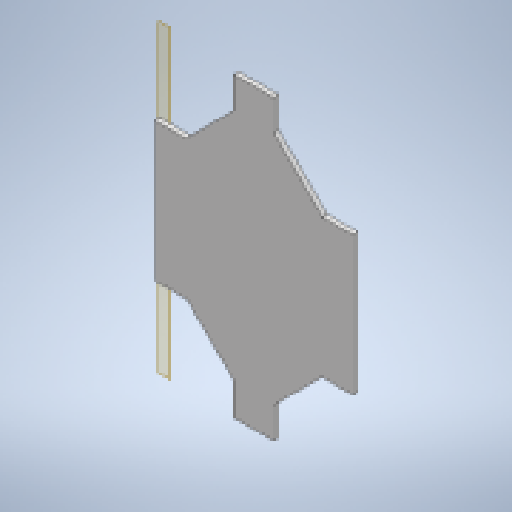
# Autodesk Inventor part: baseplate
Saved by Autodesk Inventor 2024 (Build 280153000, 153)
## iProperties
Created: 2024-01-06
Part Number: baseplate
Material: Generic
Document SubType Name: Modeling
Designer: student
Density: 1 g/cm^3
Appearance: Default
Author: student
Autodesk Inventor part; units mm, degrees
ref_plane "YZ Plane" through (0, 0, 0) normal (1, 0, 0) x (0, 1, 0)
ref_plane "XZ Plane" through (0, 0, 0) normal (0, 1, 0) x (-1, 0, 0)
ref_plane "XY Plane" through (0, 0, 0) normal (0, 0, 1) x (1, 0, 0)
ref_plane "Work Plane1" through (0, 0, 0) normal (0, 0, 1) x (1, 0, 0)
sketch "Sketch1" plane through (0, 0, 0) normal (0, 0, 1) x (1, 0, 0)
  circle A0 centre (495.3, 317.5) radius 1.5875
  circle A1 centre (495.3, 698.5) radius 1.5875
  circle A2 centre (495.3, 673.1) radius 1.5875
  circle A3 centre (495.3, 647.7) radius 1.5875
  circle A4 centre (495.3, 622.3) radius 1.5875
  circle A5 centre (495.3, 596.9) radius 1.5875
  circle A6 centre (495.3, 571.5) radius 1.5875
  circle A7 centre (495.3, 546.1) radius 1.5875
  circle A8 centre (495.3, 520.7) radius 1.5875
  circle A9 centre (495.3, 495.3) radius 1.5875
  circle A10 centre (495.3, 469.9) radius 1.5875
  circle A11 centre (495.3, 444.5) radius 1.5875
  circle A12 centre (495.3, 419.1) radius 1.5875
  circle A13 centre (495.3, 393.7) radius 1.5875
  circle A14 centre (495.3, 368.3) radius 1.5875
  circle A15 centre (495.3, 342.9) radius 1.5875
  circle A16 centre (495.3, 317.5) radius 1.5875
  circle A17 centre (495.3, 292.1) radius 1.5875
  circle A18 centre (495.3, 266.7) radius 1.5875
  circle A19 centre (495.3, 241.3) radius 1.5875
  circle A20 centre (495.3, 215.9) radius 1.5875
  circle A21 centre (495.3, 190.5) radius 1.5875
  circle A22 centre (495.3, 165.1) radius 1.5875
  circle A23 centre (495.3, 139.7) radius 1.5875
  circle A24 centre (495.3, 114.3) radius 1.5875
  circle A25 centre (495.3, 88.9) radius 1.5875
  circle A26 centre (495.3, 63.5) radius 1.5875
  circle A27 centre (495.3, 38.1) radius 1.5875
  circle A28 centre (495.3, 12.7) radius 1.5875
  line L0 (482.6, 0) -> (508, 0)
  line L1 (508, 0) -> (508, 711.2)
  line L2 (482.6, 711.2) -> (508, 711.2)
  line L3 (482.6, 0) -> (482.6, 711.2)
  circle A29 centre (469.9, 723.9) radius 1.5875
  circle A30 centre (444.5, 723.9) radius 1.5875
  circle A31 centre (419.1, 723.9) radius 1.5875
  circle A32 centre (393.7, 723.9) radius 1.5875
  circle A33 centre (368.3, 723.9) radius 1.5875
  circle A34 centre (342.9, 723.9) radius 1.5875
  circle A35 centre (317.5, 723.9) radius 1.5875
  circle A36 centre (292.1, 723.9) radius 1.5875
  circle A37 centre (266.7, 723.9) radius 1.5875
  circle A38 centre (241.3, 723.9) radius 1.5875
  circle A39 centre (215.9, 723.9) radius 1.5875
  circle A40 centre (190.5, 723.9) radius 1.5875
  circle A41 centre (165.1, 723.9) radius 1.5875
  circle A42 centre (139.7, 723.9) radius 1.5875
  circle A43 centre (114.3, 723.9) radius 1.5875
  circle A44 centre (88.9, 723.9) radius 1.5875
  circle A45 centre (63.5, 723.9) radius 1.5875
  circle A46 centre (38.1, 723.9) radius 1.5875
  line L4 (25.4, 736.6) -> (25.4, 711.2)
  line L5 (25.4, 711.2) -> (482.6, 711.2)
  line L6 (482.6, 736.6) -> (482.6, 711.2)
  line L7 (25.4, 736.6) -> (482.6, 736.6)
  circle A47 centre (38.1, -12.7) radius 1.5875
  circle A48 centre (63.5, -12.7) radius 1.5875
  circle A49 centre (88.9, -12.7) radius 1.5875
  circle A50 centre (114.3, -12.7) radius 1.5875
  circle A51 centre (139.7, -12.7) radius 1.5875
  circle A52 centre (165.1, -12.7) radius 1.5875
  circle A53 centre (190.5, -12.7) radius 1.5875
  circle A54 centre (215.9, -12.7) radius 1.5875
  circle A55 centre (241.3, -12.7) radius 1.5875
  circle A56 centre (266.7, -12.7) radius 1.5875
  circle A57 centre (292.1, -12.7) radius 1.5875
  circle A58 centre (317.5, -12.7) radius 1.5875
  circle A59 centre (342.9, -12.7) radius 1.5875
  circle A60 centre (368.3, -12.7) radius 1.5875
  circle A61 centre (393.7, -12.7) radius 1.5875
  circle A62 centre (419.1, -12.7) radius 1.5875
  circle A63 centre (444.5, -12.7) radius 1.5875
  circle A64 centre (469.9, -12.7) radius 1.5875
  line L8 (482.6, -25.4) -> (482.6, 0)
  line L9 (482.6, 0) -> (25.4, 0)
  line L10 (25.4, -25.4) -> (25.4, 0)
  line L11 (482.6, -25.4) -> (25.4, -25.4)
  circle A65 centre (12.7, 698.5) radius 1.5875
  circle A66 centre (12.7, 673.1) radius 1.5875
  circle A67 centre (12.7, 647.7) radius 1.5875
  circle A68 centre (12.7, 622.3) radius 1.5875
  circle A69 centre (12.7, 596.9) radius 1.5875
  circle A70 centre (12.7, 571.5) radius 1.5875
  circle A71 centre (12.7, 546.1) radius 1.5875
  circle A72 centre (12.7, 520.7) radius 1.5875
  circle A73 centre (12.7, 495.3) radius 1.5875
  circle A74 centre (12.7, 469.9) radius 1.5875
  circle A75 centre (12.7, 444.5) radius 1.5875
  circle A76 centre (12.7, 419.1) radius 1.5875
  circle A77 centre (12.7, 393.7) radius 1.5875
  circle A78 centre (12.7, 368.3) radius 1.5875
  circle A79 centre (12.7, 342.9) radius 1.5875
  circle A80 centre (12.7, 317.5) radius 1.5875
  circle A81 centre (12.7, 292.1) radius 1.5875
  circle A82 centre (12.7, 266.7) radius 1.5875
  circle A83 centre (12.7, 241.3) radius 1.5875
  circle A84 centre (12.7, 215.9) radius 1.5875
  circle A85 centre (12.7, 190.5) radius 1.5875
  circle A86 centre (12.7, 165.1) radius 1.5875
  circle A87 centre (12.7, 139.7) radius 1.5875
  circle A88 centre (12.7, 114.3) radius 1.5875
  circle A89 centre (12.7, 88.9) radius 1.5875
  circle A90 centre (12.7, 63.5) radius 1.5875
  circle A91 centre (12.7, 38.1) radius 1.5875
  circle A92 centre (12.7, 12.7) radius 1.5875
  line L12 (0, 0) -> (25.4, 0)
  line L13 (25.4, 0) -> (25.4, 711.2)
  line L14 (0, 711.2) -> (25.4, 711.2)
  line L15 (0, 0) -> (0, 711.2)
  line L16 (0, 533.4) -> (0, 177.8)
  line L17 (508, 177.8) -> (508, 533.4)
  line L18 (304.8, 736.6) -> (203.2, 736.6)
  line L19 (203.2, -25.4) -> (304.8, -25.4)
  line L20 (428.9731, 177.8) -> (304.8, 53.6269)
  spline S0 degree 3 number of poles 75
  line L21 (429.7528, 155.0822) -> (327.5178, 52.8472)
  line L22 (82.5441, 177.8) -> (203.2, 57.1441)
  line L23 (180.4822, 52.8472) -> (78.2472, 155.0822)
  line L24 (203.2, 656.5375) -> (80.0625, 533.4)
  line L25 (78.2472, 556.1178) -> (180.4822, 658.3528)
  line L26 (327.5178, 658.3528) -> (429.7528, 556.1178)
  line L27 (304.8, 658.3528) -> (429.7528, 533.4)
  line L28 (203.2, 736.6) -> (203.2, 656.5375)
  line L29 (203.2, 57.1441) -> (203.2, -25.4)
  line L30 (304.8, 658.3528) -> (304.8, 736.6)
  line L31 (508, 533.4) -> (429.7528, 533.4)
  line L32 (80.0625, 533.4) -> (0, 533.4)
  line L33 (0, 177.8) -> (82.5441, 177.8)
  line L34 (428.9731, 177.8) -> (508, 177.8)
  line L35 (304.8, -25.4) -> (304.8, 53.6269)
  constraints: 32 end point, 14 parallel, 4 perpendicular, 4 point on line, 3 horizontal
extrude "Extrusion1" add sketch "Sketch1" along normal blind 12.7 contours A0 | A8 | A9 | A10 | A11 | A12 | A13 | A14 | A15 | A17 | A18 | A19 | A20 | A21 | L34 L20 L35 L9 L29 L22 L33 L13 L32 L24 L28 L5 L30 L27 L31 L3 | L3 L31 L1 L34 | L35 L11 L29 L9 | L5 L28 L7 L30 | L33 L15 L32 L13 | A36 | A37 | A38 | A39 | A54 | A55 | A56 | A57 | A72 | A73 | A74 | A75 | A76 | A77 | A78 | A79 | A80 | A81 | A82 | A83 | A84 | A85
sketch "Sketch2" plane through (0, 0, 0) normal (0, 0, -1) x (-1, 0, 0)
  circle A0 centre (-495.3, 190.5) radius 1.5875 projected
  circle A1 centre (-495.3, 215.9) radius 1.5875 projected
  circle A2 centre (-495.3, 241.3) radius 1.5875 projected
  circle A3 centre (-495.3, 266.7) radius 1.5875 projected
  circle A4 centre (-495.3, 292.1) radius 1.5875 projected
  circle A5 centre (-495.3, 317.5) radius 1.5875 projected
  circle A6 centre (-495.3, 342.9) radius 1.5875 projected
  circle A7 centre (-495.3, 368.3) radius 1.5875 projected
  circle A8 centre (-495.3, 393.7) radius 1.5875 projected
  circle A9 centre (-495.3, 419.1) radius 1.5875 projected
  circle A10 centre (-495.3, 444.5) radius 1.5875 projected
  circle A11 centre (-495.3, 469.9) radius 1.5875 projected
  circle A12 centre (-495.3, 495.3) radius 1.5875 projected
  circle A13 centre (-495.3, 520.7) radius 1.5875 projected
  circle A14 centre (-215.9, 723.9) radius 1.5875 projected
  circle A15 centre (-241.3, 723.9) radius 1.5875 projected
  circle A16 centre (-266.7, 723.9) radius 1.5875 projected
  circle A17 centre (-292.1, 723.9) radius 1.5875 projected
  circle A18 centre (-12.7, 520.7) radius 1.5875 projected
  circle A19 centre (-12.7, 495.3) radius 1.5875 projected
  circle A20 centre (-12.7, 469.9) radius 1.5875 projected
  circle A21 centre (-12.7, 444.5) radius 1.5875 projected
  circle A22 centre (-12.7, 419.1) radius 1.5875 projected
  circle A23 centre (-12.7, 393.7) radius 1.5875 projected
  circle A24 centre (-12.7, 368.3) radius 1.5875 projected
  circle A25 centre (-12.7, 342.9) radius 1.5875 projected
  circle A26 centre (-12.7, 317.5) radius 1.5875 projected
  circle A27 centre (-12.7, 292.1) radius 1.5875 projected
  circle A28 centre (-12.7, 266.7) radius 1.5875 projected
  circle A29 centre (-12.7, 241.3) radius 1.5875 projected
  circle A30 centre (-12.7, 215.9) radius 1.5875 projected
  circle A31 centre (-12.7, 190.5) radius 1.5875 projected
  circle A32 centre (-215.9, -12.7) radius 1.5875 projected
  circle A33 centre (-241.3, -12.7) radius 1.5875 projected
  circle A34 centre (-266.7, -12.7) radius 1.5875 projected
  circle A35 centre (-292.1, -12.7) radius 1.5875 projected
  point P0 (0, 0)
extrude "Extrusion2" cut sketch "Sketch2" against normal blind 12.7
body "Solid1"
